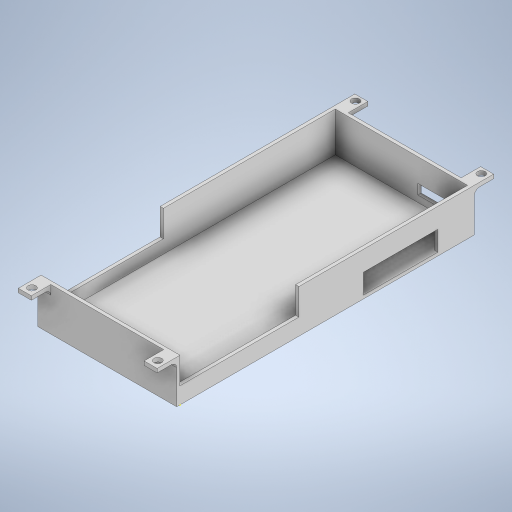
# Autodesk Inventor part: bms_mount
Saved by Autodesk Inventor 2024.2 (Build 282272000, 272)
## iProperties
Created: 2023-11-29
Part Number: bms_mount
Material: Generic
Document SubType Name: Modeling
Designer: gavin
Density: 1 g/cm^3
Appearance: Default
Author: gavin
Autodesk Inventor part; units mm, degrees
ref_plane "YZ Plane" through (0, 0, 0) normal (1, 0, 0) x (0, 1, 0)
ref_plane "XZ Plane" through (0, 0, 0) normal (0, 1, 0) x (-1, 0, 0)
ref_plane "XY Plane" through (0, 0, 0) normal (0, 0, 1) x (1, 0, 0)
sketch "Sketch1" plane through (0, 0, 0) normal (0, 1, 0) x (-1, 0, 0)
  line L0 (0, 0) -> (-101.6, 0)
  line L1 (-101.6, 0) -> (-101.6, -223.52)
  line L2 (-101.6, -223.52) -> (0, -223.52)
  line L3 (0, -223.52) -> (0, 0)
  dimension "d0" = 101.6
  dimension "d1" = 223.52
  constraints: 8 end point, 2 parallel, 1 horizontal, 1 perpendicular
  measures "d0" distance of L2.end L1.end
  measures "d1" distance of L1.end L0.end
extrude "Extrusion1" add sketch "Sketch1" along normal blind 2.54
sketch "Sketch2" plane through (0, 0, 0) normal (0, -1, 0) x (1, 0, 0)
  line L0 (104.14, 2.54) -> (-2.54, 2.54)
  line L1 (-2.54, 2.54) -> (-2.54, -226.06)
  line L2 (-2.54, -226.06) -> (104.14, -226.06)
  line L3 (104.14, -226.06) -> (104.14, 2.54)
  line L4 (101.6, 0) -> (101.6, -223.52) projected
  line L5 (0, -223.52) -> (0, 0) projected
  line L6 (101.6, -223.52) -> (0, -223.52) projected
  line L7 (0, 0) -> (101.6, 0) projected
  dimension "d4" = 2.54
  dimension "d5" = 2.54
  dimension "d6" = 2.54
  dimension "d7" = 2.54
  constraints: 8 end point, 2 parallel, 1 horizontal, 1 perpendicular
  measures "d4" distance between parallel lines of L4 L3
  measures "d5" distance between parallel lines of L5 L1
  measures "d6" distance between parallel lines of L2 L6
  measures "d7" distance between parallel lines of L7 L0
extrude "Extrusion2" add sketch "Sketch2" against normal blind 33.02
sketch "Sketch3" plane through (104.14, 0, 2.54) normal (1, 0, 0) x (0, 0, -1)
  line L0 (2.54, 2.54) -> (2.54, 33.02) projected
  line L1 (2.54, 33.02) -> (93.98, 33.02)
  line L2 (93.98, 33.02) -> (93.98, 12.7)
  line L3 (93.98, 12.7) -> (2.54, 12.7)
  line L4 (2.54, 12.7) -> (2.54, 33.02)
  point P0 (2.54, 0)
  point P1 (2.54, 12.7)
  dimension "d10" = 91.44
  dimension "d11" = 20.32
  constraints: 8 end point, 2 parallel, 1 horizontal, 1 perpendicular
  measures "d10" distance of L2.end L3.end
  measures "d11" distance of L1.end L2.end
extrude "Extrusion3" cut sketch "Sketch3" against normal up to surface (106.68 mm away)
sketch "Sketch4" plane through (104.14, 0, -226.06) normal (0, 0, -1) x (-1, 0, 0)
  line L0 (2.54, 2.54) -> (2.54, 12.7) projected
  line L1 (2.54, 2.54) -> (40.64, 2.54)
  line L2 (40.64, 2.54) -> (40.64, 15.24)
  line L3 (40.64, 15.24) -> (2.54, 15.24)
  line L4 (2.54, 15.24) -> (2.54, 2.54)
  point P0 (104.14, 0)
  point P1 (2.54, 7.62)
  dimension "d14" = 38.1
  dimension "d17" = 12.7
  constraints: 8 end point, 2 parallel, 1 horizontal, 1 perpendicular
  measures "d14" distance of L3.end L2.end
  measures "d17" distance of L1.end L2.end
extrude "Extrusion4" cut sketch "Sketch4" against normal up to surface (2.54 mm away)
sketch "Sketch5" plane through (0, 33.02, 0) normal (0, 1, 0) x (1, 0, 0)
  line L0 (104.14, -2.54) -> (-2.54, -2.54) projected
  line L1 (50.8, -2.54) -> (50.8, -16.5675)
  line L2 (114.0141, 111.76) -> (126.7141, 111.76)
  line L3 (-2.54, -2.54) -> (7.46, -2.54)
  line L4 (7.46, -2.54) -> (7.46, -17.54)
  line L5 (7.46, -17.54) -> (-2.54, -17.54)
  line L6 (-2.54, -17.54) -> (-2.54, -2.54)
  line L7 (-2.54, -2.54) -> (104.14, -2.54)
  line L8 (104.14, -2.54) -> (94.14, -2.54)
  line L9 (94.14, -2.54) -> (94.14, -17.54)
  line L10 (94.14, -17.54) -> (104.14, -17.54)
  line L11 (104.14, -17.54) -> (104.14, -2.54)
  line L12 (104.14, 226.06) -> (-2.54, 226.06)
  line L13 (7.46, 226.06) -> (7.46, 241.06)
  line L14 (7.46, 241.06) -> (-2.54, 241.06)
  line L15 (-2.54, 241.06) -> (-2.54, 226.06)
  line L16 (94.14, 226.06) -> (94.14, 241.06)
  line L17 (104.14, 241.06) -> (104.14, 226.06)
  line L18 (94.14, 241.06) -> (104.14, 241.06)
  point P0 (0, 0)
  dimension "d21" = 10
  dimension "d22" = 15
  constraints: 36 end point, 14 symmetric about line, 2 horizontal, 2 parallel, 1 midpoint, 1 perpendicular, 1 vertical
  measures "d21" distance of L4.end L5.end
  measures "d22" distance of L3.end L4.end
extrude "Extrusion5" add sketch "Sketch5" against normal blind 3
fillet "Fillet1" radius 4 4 edges at (99.14, 30.02, 2.54) (2.46, 30.02, 2.54) (2.46, 30.02, -226.06) (99.14, 30.02, -226.06)
sketch "Sketch6" plane through (104.14, 0, 2.54) normal (1, 0, 0) x (0, 0, -1)
  point P0 (2.54, 0)
sketch "Sketch7" plane through (104.14, 0, 2.54) normal (1, 0, 0) x (0, 0, -1)
  line L0 (226.06, 2.54) -> (226.06, 15.24) projected
  line L1 (226.06, 2.54) -> (143.51, 2.54)
  line L2 (143.51, 2.54) -> (143.51, 17.78)
  line L3 (143.51, 17.78) -> (226.06, 17.78)
  line L4 (226.06, 17.78) -> (226.06, 2.54)
  point P0 (2.54, 0)
  dimension "d26" = 82.55
  dimension "d27" = 15.24
  constraints: 8 end point, 2 parallel, 1 horizontal, 1 perpendicular
  measures "d26" distance of L2.end L3.end
  measures "d27" distance of L1.end L2.end
extrude "Extrusion6" cut sketch "Sketch7" against normal up to surface (2.54 mm away)
sketch "Sketch8" plane through (0, 33.02, -223.52) normal (0, 0, 1) x (1, 0, 0)
  line L0 (63.5, -30.48) -> (63.5, -17.78) projected
  line L1 (63.5, -17.78) -> (101.6, -17.78) projected
  line L2 (101.6, -30.48) -> (101.6, -17.78) projected
  line L3 (104.14, -30.48) -> (101.6, -30.48) projected
  line L4 (104.14, -15.24) -> (104.14, -30.48) projected
  line L5 (104.14, -15.24) -> (101.6, -15.24) projected
  line L6 (101.6, -15.24) -> (101.6, 0) projected
  line L7 (0, 0) -> (101.6, 0) projected
  line L8 (0, -30.48) -> (0, 0) projected
  line L9 (63.5, -30.48) -> (0, -30.48) projected
  line L10 (104.14, -30.48) -> (101.6, -30.48)
  line L11 (101.6, -30.48) -> (101.6, -15.24)
  line L12 (101.6, -15.24) -> (104.14, -15.24)
  line L13 (104.14, -15.24) -> (104.14, -30.48)
  point P0 (0, -33.02)
  constraints: 8 end point, 2 parallel, 1 horizontal, 1 perpendicular
extrude "Extrusion7" add sketch "Sketch8" along normal blind 25.4 contours L11 L5 L4 L3 L2
sketch "Sketch9" plane through (0, 2.54, 0) normal (0, 1, 0) x (1, 0, 0)
  line L0 (63.5, 226.06) -> (63.5, 223.52) projected
  line L1 (101.6474, 226.008) -> (63.5, 226.008)
  line L2 (63.5, 226.008) -> (63.5, 223.52)
  line L3 (63.5, 223.52) -> (101.6474, 223.52)
  line L4 (101.6474, 223.52) -> (101.6474, 226.008)
  point P0 (0, 0)
  constraints: 8 end point, 2 parallel, 1 horizontal, 1 perpendicular
extrude "Extrusion8" add sketch "Sketch9" along normal blind 5.08
sketch "Sketch10" plane through (0, 30.02, 0) normal (0, -1, 0) x (1, 0, 0)
  line L0 (-2.54, 17.54) -> (7.46, 17.54) projected
  line L1 (2.46, 17.54) -> (2.46, 6.54)
  line L2 (7.46, 6.54) -> (-2.54, 6.54) projected
  line L3 (7.46, 6.54) -> (7.46, 17.54) projected
  line L4 (7.46, 12.04) -> (-2.54, 12.04)
  line L5 (-2.54, 0) -> (-2.54, 17.54) projected
  point P0 (0, 0)
  point P1 (2.46, 12.04)
  constraints: 4 end point, 4 midpoint, 1 perpendicular, 1 point on line
hole "Hole1" at (2.46, 30.02, 12.04) direction (0, 1, 0) diameter 6 depth 3
pattern_linear "Rectangular Pattern1" count 2 spacing 96.68 along (1, 0, 0) count 2 spacing 248.5974 along (0, 0, -1) of "Hole1"
equation "\"d2\" = wallThickness"
equation "\"d4\" = wallThickness"
equation "\"d5\" = wallThickness"
equation "\"d6\" = wallThickness"
equation "\"d7\" = wallThickness"
equation "\"wallThickness\" = 2.54"
body "Solid1"
